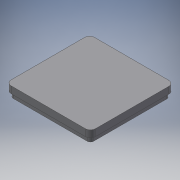
# Autodesk Inventor part: case_pantalla_3_sup
Saved by Autodesk Inventor 2019 (Build 230136000, 136)
## iProperties
Created: 2018-11-28
Part Number: case_pantalla_3_sup
Material: Steel, Mild, Welded
Document SubType Name: Modeling
Designer: cadcae
Density: 7.85 g/cm^3
Appearance: Default
Author: cadcae
Autodesk Inventor part; units mm, degrees
ref_plane "YZ Plane" through (0, 0, 0) normal (1, 0, 0) x (0, 1, 0)
ref_plane "XZ Plane" through (0, 0, 0) normal (0, 1, 0) x (-1, 0, 0)
ref_plane "XY Plane" through (0, 0, 0) normal (0, 0, 1) x (1, 0, 0)
sketch "Sketch1" plane through (0, 0, 0) normal (0, 1, 0) x (-1, 0, 0)
  line L0 (24.65, 24.4) -> (-24.65, 24.4)
  line L1 (-24.65, 24.4) -> (-24.65, -24.4)
  line L2 (-24.65, -24.4) -> (24.65, -24.4)
  line L3 (24.65, -24.4) -> (24.65, 24.4)
  line L4 (24.65, 24.4) -> (-24.65, -24.4) construction
  line L5 (-24.65, 24.4) -> (24.65, -24.4) construction
  point P0 (0, 0)
  dimension "d0" = 48.8
  dimension "d1" = 49.3
  constraints: 12 end point, 2 midpoint, 2 parallel, 1 horizontal, 1 perpendicular
  measures "d0" distance of L1.end L0.end
  measures "d1" distance of L1.end L2.end
extrude "Extrusion1" add sketch "Sketch1" along normal blind 4
fillet "Fillet1" radius 3 4 edges at (24.65, 2, 24.4) (24.65, 2, -24.4) (-24.65, 2, -24.4) (-24.65, 2, 24.4)
shell "Shell1" thickness 2.4 removed faces 1 at (7.2167, 0, -8.1333)
sketch "Sketch2" plane through (0, 0, 0) normal (0, -1, 0) x (1, 0, 0)
  arc A0 (-22.25, -21.4) -> (-21.65, -22) centre (-21.65, -21.4) ccw projected
  line L0 (-22.25, -21.4) -> (-22.25, 21.4) projected
  arc A1 (-21.65, 22) -> (-22.25, 21.4) centre (-21.65, 21.4) ccw projected
  line L1 (-21.65, 22) -> (21.65, 22) projected
  arc A2 (22.25, 21.4) -> (21.65, 22) centre (21.65, 21.4) ccw projected
  line L2 (22.25, 21.4) -> (22.25, -21.4) projected
  arc A3 (21.65, -22) -> (22.25, -21.4) centre (21.65, -21.4) ccw projected
  line L3 (21.65, -22) -> (-21.65, -22) projected
  arc A4 (-21.65, 24.4) -> (-24.65, 21.4) centre (-21.65, 21.4) ccw projected
  line L4 (-24.65, -21.4) -> (-24.65, 21.4) projected
  arc A5 (-24.65, -21.4) -> (-21.65, -24.4) centre (-21.65, -21.4) ccw projected
  line L5 (21.65, -24.4) -> (-21.65, -24.4) projected
  arc A6 (21.65, -24.4) -> (24.65, -21.4) centre (21.65, -21.4) ccw projected
  line L6 (24.65, 21.4) -> (24.65, -21.4) projected
  arc A7 (24.65, 21.4) -> (21.65, 24.4) centre (21.65, 21.4) ccw projected
  line L7 (-21.65, 24.4) -> (21.65, 24.4) projected
  line L8 (21.65, 23.2) -> (-21.65, 23.2)
  arc A8 (-21.65, 23.2) -> (-23.45, 21.4) centre (-21.65, 21.4) ccw
  line L9 (-23.45, 21.4) -> (-23.45, -21.4)
  arc A9 (-23.45, -21.4) -> (-21.65, -23.2) centre (-21.65, -21.4) ccw
  line L10 (-21.65, -23.2) -> (21.65, -23.2)
  arc A10 (21.65, -23.2) -> (23.45, -21.4) centre (21.65, -21.4) ccw
  line L11 (23.45, -21.4) -> (23.45, 21.4)
  arc A11 (23.45, 21.4) -> (21.65, 23.2) centre (21.65, 21.4) ccw
  point P0 (0, 0)
  dimension "d6" = 1.2
  constraints: 8 end point, 8 point on circle, 4 centre point, 7 other
  measures "d6" distance between parallel lines of L1 L8
extrude "Extrusion2" add sketch "Sketch2" along normal blind 3 contours A11 L11 A10 L10 A9 L9 A8 L8
sketch "Sketch3" plane through (0, 0, 0) normal (0, 0, 1) x (1, 0, 0)
  point P0 (0, 0)
body "Solid1"
